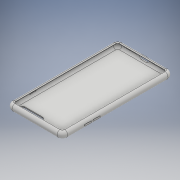
# Autodesk Inventor part: case
Saved by Autodesk Inventor 2017 (Build 210142000, 142)
## iProperties
Created: 2016-11-03
Part Number: case
Material: Generic
Document SubType Name: Modeling
Designer: skutz
Density: 1 g/cm^3
Appearance: Default
Author: skutz
Autodesk Inventor part; units mm, degrees
sketch "Sketch1" plane through (0, 0, 0) normal (0, 0, 1) x (1, 0, 0)
  line L0 (0, 0) -> (77.94, 0)
  line L1 (77.94, 0) -> (77.94, 158.22)
  line L2 (77.94, 158.22) -> (0, 158.22)
  line L3 (0, 158.22) -> (0, 0)
  dimension "d0" = 77.94
  dimension "d1" = 158.22
  constraints: 8 end point, 2 parallel, 1 horizontal, 1 perpendicular
  measures "d0" distance of L2.end L1.end
  measures "d1" distance of L1.end L0.end
extrude "Extrusion1" add sketch "Sketch1" along normal mid plane 7.3
fillet "Fillet1" radius 6.28 4 edges at (0, 0, 0) (77.94, 0, 0) (77.94, 158.22, 0) (0, 158.22, 0)
fillet "Fillet2" radius 3.65 16 edges at (1.8394, 156.3806, -3.65) (38.97, 158.22, -3.65) (76.1006, 156.3806, -3.65) (77.94, 79.11, -3.65) (76.1006, 1.8394, -3.65) (38.97, 0, -3.65) (1.8394, 1.8394, -3.65) (0, 79.11, -3.65) (1.8394, 1.8394, 3.65) (38.97, 0, 3.65) (76.1006, 1.8394, 3.65) (77.94, 79.11, 3.65) (76.1006, 156.3806, 3.65) (38.97, 158.22, 3.65) (1.8394, 156.3806, 3.65) (0, 79.11, 3.65)
shell "Shell1" thickness 1.5 outward yes removed faces 1 at (27.1966, 103.3867, 3.65)
sketch "Sketch2" plane through (0, 0, -5.15) normal (0, 0, -1) x (-1, 0, 0)
  line L0 (-79.44, 151.94) -> (-79.44, 6.28) construction
  arc A0 (-79.44, 6.28) -> (-71.66, -1.5) centre (-71.66, 6.28) ccw construction
  line L1 (-71.66, -1.5) -> (-6.28, -1.5) construction
  arc A1 (-6.28, -1.5) -> (1.5, 6.28) centre (-6.28, 6.28) ccw construction
  line L2 (1.5, 6.28) -> (1.5, 151.94) construction
  arc A2 (1.5, 151.94) -> (-6.28, 159.72) centre (-6.28, 151.94) ccw construction
  line L3 (-6.28, 159.72) -> (-71.66, 159.72) construction
  arc A3 (-71.66, 159.72) -> (-79.44, 151.94) centre (-71.66, 151.94) ccw construction
  line L4 (-9.3832, 9.3332) -> (-34.3832, 9.3332) construction
  line L5 (-9.3832, 14.3332) -> (-34.3832, 14.3332)
  line L6 (-34.3832, 4.3332) -> (-9.3832, 4.3332)
  arc A4 (-9.3832, 4.3332) -> (-9.3832, 14.3332) centre (-9.3832, 9.3332) ccw
  arc A5 (-34.3832, 14.3332) -> (-34.3832, 4.3332) centre (-34.3832, 9.3332) ccw
  point P0 (0, 0)
  point P1 (-14.155, 9.3332)
  point P2 (-21.058, 5.5966)
  point P3 (-21.8832, 9.3332)
  dimension "d68" = 25
  dimension "d69" = 10
  dimension "d70" = 35
  constraints: 8 end point, 4 point on circle, 4 tangent, 2 centre point, 1 horizontal, 1 midpoint, 1 parallel
  measures "d68" distance of L4.start L4.end
  measures "d69" diameter of A5
extrude "Extrusion2" cut sketch "Sketch2" against normal blind 7.3
ref_plane "Work Plane1" through (79.44, 39.555, 0) normal (1, 0, 0) x (0, 1, 0)
ref_plane "Work Plane2" through (-1.5, 118.665, 0) normal (1, 0, 0) x (0, 1, 0)
ref_plane "Work Plane3" through (58.455, 159.72, 0) normal (0, 1, 0) x (-1, 0, 0)
ref_plane "Work Plane4" through (38.97, 39.555, 0) normal (1, 0, 0) x (0, 1, 0)
sketch "Sketch4" plane through (58.455, 159.72, 0) normal (0, 1, 0) x (-1, 0, 0)
  line L0 (12.66, 0.35) -> (26.31, 0.35) construction
  line L1 (15.66, -2.65) -> (23.31, -2.65)
  line L2 (23.31, 3.35) -> (15.66, 3.35)
  arc A0 (15.66, 3.35) -> (15.66, -2.65) centre (15.66, 0.35) ccw
  arc A1 (23.31, -2.65) -> (23.31, 3.35) centre (23.31, 0.35) ccw
  arc A2 (54.805, -5.15) -> (54.805, 5.15) centre (54.805, 0) ccw construction
  arc A3 (54.805, -5.15) -> (54.805, 5.15) centre (54.805, 0) ccw projected
  circle A4 centre (-9.045, 0.35) radius 1
  line L3 (52.175, -3.65) -> (54.805, -3.65) projected
  line L4 (54.805, -3.65) -> (52.175, -3.65) projected
  line L5 (52.175, -3.65) -> (-13.205, -3.65) projected
  line L6 (-13.205, -3.65) -> (-15.835, -3.65) projected
  line L7 (-15.835, -3.65) -> (-13.205, -3.65) projected
  line L8 (-13.205, -3.65) -> (52.175, -3.65) projected
  line L9 (-13.205, -5.15) -> (52.175, -5.15) projected
  line L10 (-20.985, -7.21) -> (-20.985, 7.21) projected
  circle A5 centre (7.455, 0.35) radius 1
  circle A6 centre (-6.685, 0.35) radius 1
  circle A7 centre (-4.325, 0.35) radius 1
  circle A8 centre (-1.965, 0.35) radius 1
  circle A9 centre (0.395, 0.35) radius 1
  circle A10 centre (2.755, 0.35) radius 1
  circle A11 centre (5.115, 0.35) radius 1
  arc A12 (-15.835, 3.65) -> (-15.835, -3.65) centre (-15.835, 0) ccw projected
  arc A13 (54.805, -3.65) -> (54.805, 3.65) centre (54.805, 0) ccw projected
  line L11 (52.175, 3.65) -> (-13.205, 3.65) projected
  line L12 (-15.835, 3.65) -> (-13.205, 3.65) projected
  line L13 (52.175, 3.65) -> (54.805, 3.65) projected
  line L14 (19.485, -7.21) -> (19.485, 7.21) projected
  circle A14 centre (48.015, 0.35) radius 1
  circle A15 centre (31.515, 0.35) radius 1
  circle A16 centre (45.655, 0.35) radius 1
  circle A17 centre (43.295, 0.35) radius 1
  circle A18 centre (40.935, 0.35) radius 1
  circle A19 centre (38.575, 0.35) radius 1
  circle A20 centre (36.215, 0.35) radius 1
  circle A21 centre (33.855, 0.35) radius 1
  point P0 (58.455, 0)
  point P1 (19.485, 0.35)
  point P2 (59.955, 0)
  point P3 (-19.485, 0)
  point P4 (58.455, 0)
  dimension "d14" = 13.65
  dimension "d15" = 6
  dimension "d18" = 2
  dimension "d19" = 4
  dimension "d20" = 4
  dimension "d22" = 2
  dimension "d24" = 4
  dimension "d27" = 2.36
  dimension "d32" = 10.44
  dimension "d33" = 26.94
  dimension "d34" = 38.97
  constraints: 18 centre point, 9 point on circle, 8 end point, 8 symmetric about line, 4 tangent, 2 horizontal, 2 point on line, 1 coincident, 1 midpoint, 1 parallel, 20 other
  measures "d14" distance of L0.start L0.end
  measures "d15" diameter of A1
  measures "d18" diameter of A4
  measures "d19" distance from line of L5 A4.centre
  measures "d20" distance between parallel lines of L5 L0
  measures "d22" diameter of A5
  measures "d24" distance from line of L5 A5.centre
  measures "d27" distance of A4.centre A6.centre
  measures "d32" horizontal distance of point (-19.485, 0) A4.centre
  measures "d33" horizontal distance of point (-19.485, 0) A5.centre
  measures "d34" horizontal distance of point (19.485, 0.35) point (-19.485, 0)
extrude "Extrusion3" cut sketch "Sketch4" against normal blind 5 contours A0 L2 L14 L1 | L14 L2 A1 L1 | A4 | A5 | A6 | A7 | A8 | A9 | A10 | A11 | A14 | A15 | A16 | A17 | A18 | A19 | A20 | A21
fillet "Fillet3" radius 1 25 edges at (4.4202, 4.4202, 5.15) (0.7787, 0.7787, -0.0001) (6.28, 0.0084, 3.6416) (6.28, 0.0084, -3.6416) (4.4202, 4.4202, -5.15) (3.6499, 79.11, 5.15) (-1.5, 79.11, 0.0001) (3.6499, 79.11, -5.15) (4.4202, 153.7998, 5.15) (0.7787, 157.4413, 0.0001) (4.4202, 153.7998, -5.15) (38.97, 154.5701, 5.15) (38.97, 154.5701, -5.15) (73.5198, 153.7998, 5.15) (73.5198, 153.7998, -5.15) (77.1613, 157.4413, 0.0001) (74.2901, 79.11, -5.15) (74.2901, 79.11, 5.15) (79.44, 79.11, 0.0001) (73.5198, 4.4202, -5.15) (73.5198, 4.4202, 5.15) (77.1613, 0.7787, 0.0001) (38.97, 3.6499, 5.15) (38.97, 3.6499, -5.15) (38.97, -1.5, -0.0001)
sketch "Sketch6" plane through (79.44, 39.555, 0) normal (1, 0, 0) x (0, 1, 0)
  line L0 (-8.315, 0) -> (0.305, 0) construction
  line L1 (-8.315, -1) -> (0.305, -1)
  line L2 (0.305, 1) -> (-8.315, 1)
  arc A0 (-8.315, 1) -> (-8.315, -1) centre (-8.315, 0) ccw
  arc A1 (0.305, -1) -> (0.305, 1) centre (0.305, 0) ccw
  line L3 (4.295, 0) -> (12.915, 0) construction
  line L4 (4.295, -1) -> (12.915, -1)
  line L5 (12.915, 1) -> (4.295, 1)
  arc A2 (4.295, 1) -> (4.295, -1) centre (4.295, 0) ccw
  arc A3 (12.915, -1) -> (12.915, 1) centre (12.915, 0) ccw
  point P0 (-39.555, 0)
  point P1 (-4.005, 0)
  point P2 (8.605, 0)
  dimension "d41" = 35.55
  dimension "d42" = 10.62
  dimension "d43" = 10.62
  dimension "d44" = 48.16
  constraints: 16 end point, 8 point on circle, 8 tangent, 4 centre point, 2 horizontal, 2 midpoint, 2 parallel, 1 horizontal alignment
  measures "d41" distance of point (-4.005, 0) point (-39.555, 0)
  measures "d44" distance of point (-39.555, 0) point (8.605, 0)
extrude "Extrusion4" add sketch "Sketch6" along normal blind 0.5
ref_plane "Work Plane6" through (77.94, 39.555, 0) normal (1, 0, 0) x (0, 1, 0)
sketch "Sketch8" plane through (77.94, 39.555, 0) normal (1, 0, 0) x (0, 1, 0)
  line L0 (-8.315, -1) -> (0.305, -1) projected
  arc A0 (0.305, -1) -> (0.305, 1) centre (0.305, 0) ccw projected
  line L1 (0.305, 1) -> (-8.315, 1) projected
  arc A1 (-8.315, 1) -> (-8.315, -1) centre (-8.315, 0) ccw projected
  line L2 (4.295, -1) -> (12.915, -1) projected
  arc A2 (12.915, -1) -> (12.915, 1) centre (12.915, 0) ccw projected
  line L3 (12.915, 1) -> (4.295, 1) projected
  arc A3 (4.295, 1) -> (4.295, -1) centre (4.295, 0) ccw projected
  point P0 (-39.555, 0)
extrude "Extrusion5" cut sketch "Sketch8" against normal blind 0.5
sketch "Sketch9" plane through (-1.5, 118.665, 0) normal (1, 0, 0) x (0, 1, 0)
  line L0 (-78.805, 0) -> (-87.425, 0) construction
  line L1 (-112.385, 3.65) -> (-112.385, -3.65) projected
  line L2 (-78.805, -1) -> (-87.425, -1)
  line L3 (-87.425, 1) -> (-78.805, 1)
  arc A0 (-78.805, -1) -> (-78.805, 1) centre (-78.805, 0) ccw
  arc A1 (-87.425, 1) -> (-87.425, -1) centre (-87.425, 0) ccw
  point P0 (-118.665, 0)
  point P1 (-83.115, 0)
  dimension "d53" = 10.62
  dimension "d54" = 2
  dimension "d55" = 35.55
  constraints: 8 end point, 4 point on circle, 4 tangent, 2 centre point, 1 midpoint, 1 parallel, 1 perpendicular
  measures "d54" distance between parallel lines of L2 L3
  measures "d55" distance of point (-118.665, 0) point (-83.115, 0)
extrude "Extrusion6" add sketch "Sketch9" against normal blind 0.5
ref_plane "Work Plane9" through (0, 118.665, 0) normal (1, 0, 0) x (0, 1, 0)
sketch "Sketch11" plane through (0, 118.665, 0) normal (1, 0, 0) x (0, 1, 0)
  line L0 (-78.805, -1) -> (-87.425, -1) projected
  arc A0 (-87.425, 1) -> (-87.425, -1) centre (-87.425, 0) ccw projected
  line L1 (-87.425, 1) -> (-78.805, 1) projected
  arc A1 (-78.805, -1) -> (-78.805, 1) centre (-78.805, 0) ccw projected
  point P0 (-118.665, 0)
extrude "Extrusion8" cut sketch "Sketch11" against normal blind 0.5 and the other way blind 0.25
body "Solid1"
